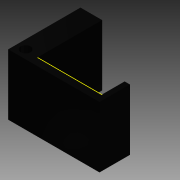
# Autodesk Inventor part: schlitten
Saved by Autodesk Inventor 2013 (Build 170138000, 138)
## iProperties
Created: 2012-10-21
Part Number: schlitten
Material: Acetalharz, schwarz
Document SubType Name: Modeling
Designer: fivef
Density: 1.425 g/cm^3
Mass: 387.859 g
Surface Area: 492.718 cm^2
Volume: 272.181 cm^3
Author: fivef
Autodesk Inventor part; units mm, degrees
ref_plane "YZ Plane" through (0, 0, 0) normal (1, 0, 0) x (0, 1, 0)
ref_plane "XZ Plane" through (0, 0, 0) normal (0, 1, 0) x (-1, 0, 0)
ref_plane "XY Plane" through (0, 0, 0) normal (0, 0, 1) x (1, 0, 0)
sketch "Skizze1" plane through (0, 0, 0) normal (0, 0, 1) x (1, 0, 0)
  line L0 (0, 0) -> (120, 0)
  line L1 (120, 0) -> (120, 40)
  line L2 (120, 40) -> (113, 40)
  line L3 (113, 40) -> (113, 10)
  line L4 (113, 10) -> (28.5, 10)
  line L5 (28.5, 10) -> (28.5, 95)
  line L6 (28.5, 95) -> (0, 95)
  line L7 (0, 95) -> (0, 0)
  circle A0 centre (11.5, 11.5) radius 6.5
  dimension "d0" = 120
  dimension "d2" = 40
  dimension "d3" = 7
  dimension "d4" = 10
  dimension "d5" = 95
  dimension "d7" = 13
  dimension "d10" = 11.5
  dimension "d11" = 11.5
  dimension "d15" = 17
  constraints: 16 end point, 5 parallel, 1 centre point, 1 coincident
  measures "d0" distance of L0.start L0.end
  measures "d2" distance of L0.end L1.end
  measures "d3" distance of L1.end L2.end
  measures "d4" distance between parallel lines of L0 L4
  measures "d5" distance of L6.end point (0, 0)
  measures "d7" diameter of A0
  measures "d10" distance from line of A0.centre L7
  measures "d11" distance from line of A0.centre L0
  measures "d15" distance from line of L5 A0.centre
extrude "Extrusion1" add sketch "Skizze1" along normal mid plane 80
sketch "Skizze2" plane through (28.5, 10, 40) normal (0, 1, 0) x (1, 0, 0)
  line L0 (0, 80) -> (0, 0) projected
  line L1 (84.5, 0) -> (0, 0) projected
  line L2 (84.5, 80) -> (84.5, 0) projected
  line L3 (0, 80) -> (84.5, 80) projected
  point P0 (-28.5, 40)
  point P1 (41.5, 40)
  point P2 (41.5, 40)
  dimension "d16" = 41.5
  constraints: 1 coincident
  measures "d16" distance from line of point (41.5, 40) L0
